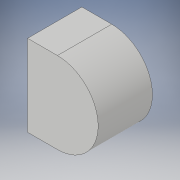
# Autodesk Inventor part: trzym2
Saved by Autodesk Inventor 2019 (Build 230136000, 136)
## iProperties
Created: 2020-01-12
Part Number: trzym2
Material: Ogólny
Document SubType Name: Modeling
Designer: Karolina
Density: 1 g/cm^3
Appearance: Domyślna
Author: Karolina
Autodesk Inventor part; units mm, degrees
ref_plane "YZ Plane" through (0, 0, 0) normal (1, 0, 0) x (0, 1, 0)
ref_plane "XZ Plane" through (0, 0, 0) normal (0, 1, 0) x (-1, 0, 0)
ref_plane "XY Plane" through (0, 0, 0) normal (0, 0, 1) x (1, 0, 0)
sketch "Szkic1" plane through (0, 0, 0) normal (0, 0, 1) x (1, 0, 0)
  line L0 (-0.26, 0) -> (1.56, 0) construction
  line L1 (0, -0.3) -> (0, 1.8) construction
  line L2 (0, 0) -> (1.3, 0)
  line L3 (1.3, 0) -> (1.3, 1.5)
  line L4 (1.3, 1.5) -> (0, 1.5)
  line L5 (0, 1.5) -> (0, 0)
  dimension "d0" = 1.5
  dimension "d1" = 1.3
  constraints: 8 end point, 2 parallel, 1 horizontal, 1 perpendicular
  measures "d0" distance of L2.end L3.end
  measures "d1" distance of L3.end L4.end
extrude "Wyciągnięcie proste1" add sketch "Szkic1" along normal blind 1
fillet "Zaokrąglenie1" radius 0.75 2 edges at (1.3, 1.5, 0.5) (1.3, 0, 0.5)
